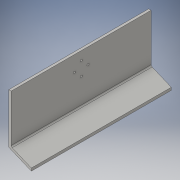
# Autodesk Inventor part: CowCatcherRearShort
Saved by Autodesk Inventor 2016 (Build 200138000, 138)
## iProperties
Created: 2016-12-19
Part Number: CowCatcherRearShort
Material: Generic
Document SubType Name: Modeling
Designer: lachesis
Density: 1 g/cm^3
Appearance: Default
Author: lachesis
Autodesk Inventor part; units mm, degrees
ref_plane "YZ Plane" through (0, 0, 0) normal (1, 0, 0) x (0, 1, 0)
ref_plane "XZ Plane" through (0, 0, 0) normal (0, 1, 0) x (-1, 0, 0)
ref_plane "XY Plane" through (0, 0, 0) normal (0, 0, 1) x (1, 0, 0)
sketch "Sketch3" plane through (0, 0, 0) normal (0, 0, 1) x (1, 0, 0)
  line L0 (-1.5, 30.2485) -> (1.5, 30.2485)
  line L1 (1.5, 30.2485) -> (1.5, -30.2485)
  line L2 (1.5, -30.2485) -> (-1.5, -30.2485)
  line L3 (-1.5, -30.2485) -> (-1.5, 30.2485)
  line L4 (1.5, -28.2515) -> (26, -38.4996)
  line L5 (26, -38.4996) -> (26, -41.7515)
  line L6 (26, -41.7515) -> (-1.5, -30.2485)
  point P0 (0, 0)
  point P1 (0, 30.2485)
  point P2 (1.5, 0)
  dimension "d20" = 3
  dimension "d26" = 24.5
  dimension "d39" = 3
  dimension "d41" = 58.5
  dimension "d43" = 72
  constraints: 14 end point, 3 parallel, 2 midpoint, 1 horizontal, 1 horizontal alignment, 1 perpendicular, 1 point on line, 1 vertical, 1 vertical alignment
  measures "d20" distance of L0.start L0.end
  measures "d26" distance between parallel lines of L5 L1
  measures "d39" distance between parallel lines of L6 L4
  measures "d41" distance of L4.start L0.end
  measures "d43" distance from line of L5.end L0
extrude "Extrusion3" add sketch "Sketch3" along normal blind 170
sketch "Sketch4" plane through (1.5, -28.2515, 0) normal (1, 0, 0) x (0, 0, -1)
  circle A0 centre (-85, 48.031) radius 1.345
  circle A1 centre (-85, 31.369) radius 1.345
  circle A2 centre (-76.669, 39.7) radius 1.345
  circle A3 centre (-93.331, 39.7) radius 1.345
  line L0 (0, 58.5) -> (0, 0) projected
  line L1 (0, 58.5) -> (-170, 58.5) projected
  line L2 (-170, 0) -> (-170, 58.5) projected
  line L3 (0, 0) -> (-170, 0) projected
  point P0 (-85, 58.5)
  dimension "d28" = 2.69
  dimension "d30" = 8.331
  dimension "d31" = 8.331
  dimension "d32" = 8.331
  dimension "d33" = 8.331
  dimension "d34" = 16.662
  dimension "d35" = 16.662
  dimension "d36" = 10.469
  constraints: 4 centre point, 3 equal radius, 1 midpoint, 1 vertical alignment
  measures "d28" diameter of A0
  measures "d30" horizontal distance of A2.centre A0.centre
  measures "d31" horizontal distance of A1.centre A3.centre
  measures "d32" horizontal distance of A0.centre A3.centre
  measures "d33" horizontal distance of A2.centre A1.centre
  measures "d34" distance of A1.centre A0.centre
  measures "d35" distance of A2.centre A3.centre
  measures "d36" distance from line of A0.centre L1
extrude "Extrusion4" cut sketch "Sketch4" against normal through all contours A0 | A1 | A2 | A3
fillet "Fillet1" radius 2 1 edges at (1.5, -28.2515, 85)
equation "\"d31\" = d30"
equation "\"d32\" = d30"
equation "\"d33\" = d30"
equation "\"d35\" = d34"
body "Solid2"
